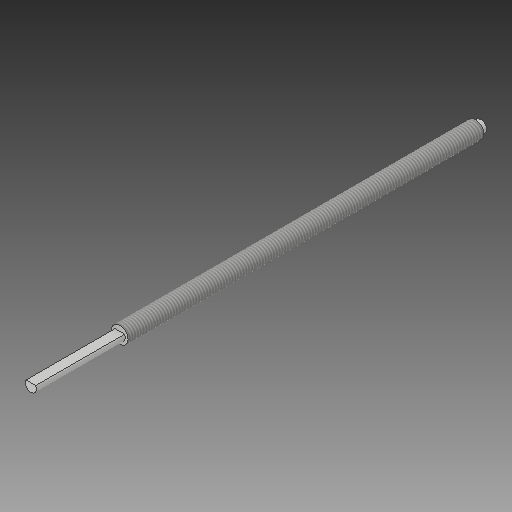
# Autodesk Inventor part: Part2
Saved by Autodesk Inventor 2019 (Build 230136000, 136)
## iProperties
Created: 2018-09-13
Part Number: Part2
Material: Generic
Document SubType Name: Modeling
Designer: drawing
Density: 1 g/cm^3
Appearance: Default
Author: drawing
Autodesk Inventor part; units mm, degrees
ref_plane "YZ Plane" through (0, 0, 0) normal (1, 0, 0) x (0, 1, 0)
ref_plane "XZ Plane" through (0, 0, 0) normal (0, 1, 0) x (-1, 0, 0)
ref_plane "XY Plane" through (0, 0, 0) normal (0, 0, 1) x (1, 0, 0)
sketch "Sketch1" plane through (0, 0, 0) normal (0, 0, 1) x (1, 0, 0)
  circle A0 centre (0, 0) radius 4.7625
  dimension "d0" = 9.525
  constraints: 1 centre point, 1 coincident
  measures "d0" diameter of A0
extrude "Extrusion1" add sketch "Sketch1" along normal mid plane 254
thread "Thread1" size "3/8-16 UNC" class "2A" standard "ANSI Unified Screw Threads" full length
sketch "Sketch2" plane through (0, 0, 127) normal (0, 0, 1) x (1, 0, 0)
  arc A0 (-2.7496, 1.5875) -> (2.7496, 1.5875) centre (0, 0) ccw
  line L0 (-2.7496, 1.5875) -> (2.7496, 1.5875)
  circle A1 centre (0, 0) radius 8.1081
  dimension "d5" = 6.35
  dimension "d6" = 1.5875
  constraints: 2 centre point, 2 coincident, 2 end point, 2 point on circle, 1 horizontal
  measures "d5" diameter of A0
  measures "d6" distance from line of point (0, 0) L0
extrude "Extrusion2" cut sketch "Sketch2" against normal blind 50.8
sketch "Sketch4" plane through (0, 0, -127) normal (0, 0, -1) x (-1, 0, 0)
  circle A0 centre (0, 0) radius 3.175
  dimension "d16" = 6.35
  constraints: 1 centre point, 1 coincident
  measures "d16" diameter of A0
extrude "Extrusion3" add sketch "Sketch4" along normal blind 3.175
body "Solid1"
